kegelstopfen_v4 (Autodesk Fusion 360 design; units mm, degrees)
Autodesk Fusion 360 part; units mm, degrees
cylinder "Grundkörper Zylinder1" add diameter 11 height 1 placed x (1, 0, 0) y (0, 0, -1) z (0, 1, 0) at (0, 0, 0)
sketch "Skizze2" plane through (0, 0, 0) normal (1, 0, 0) x (0, 0, -1)
  line L0 (0, 1) -> (0, 10)
  line L1 (0, 10) -> (3.6, 10)
  line L2 (0, 1) -> (3.85, 1)
  line L3 (3.85, 1) -> (3.6, 10)
  dimension "d3" = 3.6
  dimension "d4" = 3.85
  dimension "d5" = 9
  constraint vertical L0
  constraint perpendicular L0 L1
  constraint perpendicular L0 L2
  measures "d3" distance of L0.end L1.end
  measures "d4" distance of L0.start L2.end
  measures "d5" distance of L0.start L0.end
revolve "Drehen1" add sketch "Skizze2" angle 360 about axis through (0, 1, 0) along (0, 1, 0)
cylinder "Grundkörper Zylinder2" cut diameter 2.5 height -23 placed x (1, 0, 0) y (0, 0, -1) z (0, 1, 0) at (0, 10, 0)
fillet "Abrundung1" radius 0.3 6 faces at (5.4727, 0.6667, 0.5476) (4.9259, 1, 0.3691) (0.21, 10, -2.8021) (1.2438, 6.6667, 0.1245) (4.0629, 0, 0.2732) (3.5528, 2.2, 1.3944)
